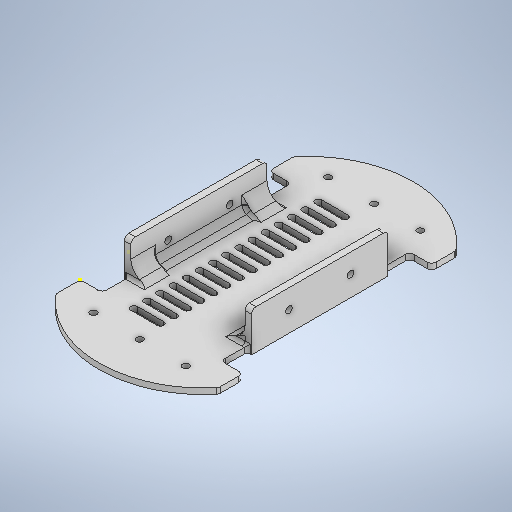
# Autodesk Inventor part: module_part2_nologo_asymmetric
Saved by Autodesk Inventor 2025.2 (Build 292293000, 293)
## iProperties
Created: 2025-05-02
Part Number: module_part2_nologo_asymmetric
Material: Generic
Document SubType Name: Modeling
Designer: holz
Density: 1 g/cm^3
Appearance: Default
Author: holz
Autodesk Inventor part; units mm, degrees
ref_plane "YZ Plane" through (0, 0, 0) normal (1, 0, 0) x (0, 1, 0)
ref_plane "XZ Plane" through (0, 0, 0) normal (0, 1, 0) x (-1, 0, 0)
ref_plane "XY Plane" through (0, 0, 0) normal (0, 0, 1) x (1, 0, 0)
sketch "Sketch1" plane through (0, 0, 0) normal (0, 1, 0) x (-1, 0, 0)
  line L0 (0, 0) -> (-74, 0)
  line L1 (-74, -86) -> (-74, -86)
  line L2 (-74, -86) -> (0, -86)
  line L3 (0, -86) -> (0, -97)
  line L4 (0, -97) -> (-74, -97)
  line L5 (-74, -97) -> (-74, -86)
  line L6 (-74, 0) -> (0, 0)
  line L7 (0, 0) -> (0, 11)
  line L8 (0, 11) -> (-74, 11)
  line L9 (-74, 11) -> (-74, 0)
  line L10 (-74, 11) -> (0, 11)
  line L11 (0, 11) -> (0, 28.5)
  line L12 (0, 28.5) -> (-74, 28.5)
  line L13 (-74, 28.5) -> (-74, 11)
  line L14 (-74, -97) -> (0, -97)
  line L15 (0, -97) -> (0, -114.5)
  line L16 (0, -114.5) -> (-74, -114.5)
  line L17 (-74, -114.5) -> (-74, -97)
  arc A0 (0, 11) -> (-74, 11) centre (-37, -19.3643) ccw
  arc A1 (-74, -97) -> (0, -97) centre (-37, -66.6357) ccw
  line L18 (-37, 0) -> (-65, 0)
  line L19 (-69, -86) -> (-39, -86)
  line L20 (-37, 0) -> (-5, 0)
  line L21 (-9, -86) -> (-39, -86)
  line L22 (-9, -86) -> (-10, -86)
  line L23 (-10, -86) -> (-10, 0)
  line L24 (-10, 0) -> (-8, 0)
  line L25 (-69, -86) -> (-66, -86)
  line L26 (-66, 0) -> (-65, 0)
  line L27 (0, 11) -> (-74, 11)
  line L28 (-74, 11) -> (-74, -49.7286)
  line L29 (-74, -49.7286) -> (0, -49.7286)
  line L30 (0, -49.7286) -> (0, 11)
  line L31 (-37, -49.7286) -> (-37, -97)
  line L32 (-37, -49.7286) -> (-37, 0)
  line L33 (-37, -97) -> (-10, -97)
  line L34 (-9, 0) -> (-37, 0)
  line L35 (-37, 0) -> (-37, -97)
  line L36 (-37, 0) -> (-64, 0)
  line L37 (-64, 0) -> (-64, -86)
  line L38 (-64, -86) -> (-37, -86)
  line L39 (-37, -86) -> (-37, 0)
  point P0 (-10, 0)
  dimension "d1" = 86
  dimension "d2" = 11
  dimension "d3" = 11
  dimension "d4" = 17.5
  dimension "d5" = 17.5
  dimension "d11" = 74
  dimension "d12" = 74
  dimension "d15" = 27
  dimension "d16" = 27
  constraints: 80 end point, 18 parallel, 12 horizontal, 8 point on line, 7 perpendicular, 6 point on circle, 5 midpoint, 2 centre point, 2 tangent, 1 collinear
  measures "d1" distance of L1.start L0.end
  measures "d2" distance of L2.end L3.end
  measures "d3" distance of L7.end L6.end
  measures "d4" distance of L11.end L10.end
  measures "d5" distance of L14.end L15.end
  measures "d11" distance of L7.end L8.end
  measures "d12" distance of L3.end L4.end
  measures "d15" distance of L23.end L36.start
  measures "d16" distance of L36.end L34.end
extrude "Extrusion1" add sketch "Sketch1" against normal blind 2.6 contours L0 L9 L8 L7 | L8 A0 | L29 L32 L0 L23 | L23 L2 L31 L29 | L2 L3 L4 L31 | L31 L2 L37 L29 | L29 L37 L0 L32 | L31 L4 L5 L2 | L4 A1
fillet "Face Fillet1" radius 2 1 edges at (74, -1.3, -86)
fillet "Face Fillet2" radius 2 1 edges at (64, -1.3, -86)
fillet "Face Fillet3" radius 2 1 edges at (74, -1.3, 11)
fillet "Face Fillet4" radius 2 1 edges at (0, -1.3, -86)
fillet "Face Fillet5" radius 2 1 edges at (0, -1.3, 11)
fillet "Face Fillet6" radius 2 1 edges at (0, -1.3, 0)
fillet "Face Fillet7" radius 2 1 edges at (0, -1.3, -97)
fillet "Face Fillet8" radius 2 1 edges at (74, -1.3, -97)
fillet "Face Fillet9" radius 2 1 edges at (74, -1.3, 0)
fillet "Face Fillet10" radius 2 1 edges at (10, -1.3, -86)
fillet "Face Fillet11" radius 2 1 edges at (10, -1.3, 0)
fillet "Face Fillet12" radius 2 1 edges at (64, -1.3, 0)
sketch "Sketch5" plane through (0, 0, 0) normal (0, 1, 0) x (1, 0, 0)
  arc A0 (10, 84) -> (8, 86) centre (8, 84) ccw projected
  line L0 (64, 2) -> (64, 84) projected
  line L1 (10, 84) -> (64, 84)
  line L2 (64, 84) -> (64, 71.4558)
  line L3 (64, 71.4558) -> (10, 71.4558)
  line L4 (10, 71.4558) -> (10, 84)
  line L5 (37, 84) -> (37, 60.4451)
  line L6 (26.2602, 84) -> (40.4168, 84)
  line L7 (40.4168, 84) -> (40.4168, 82.5)
  line L8 (40.4168, 82.5) -> (26.2602, 82.5)
  line L9 (26.2602, 82.5) -> (26.2602, 84)
  line L10 (8, 86) -> (2, 86) projected
  line L11 (2, 86) -> (74.2134, 86)
  line L12 (70.1915, 96.9) -> (-2.0219, 96.9)
  line L13 (70.1915, 96.9) -> (-4.0219, 96.9)
  line L14 (-4.0219, 96.9) -> (-4.0219, 86)
  line L15 (-4.0219, 86) -> (70.1915, 86)
  line L16 (74, 96.2758) -> (74, 88) projected
  line L17 (74, 88) -> (74, 85.5591)
  line L18 (74, 85.5591) -> (74, 96.9)
  line L19 (37, 84) -> (37, 116.0596)
  line L20 (37, 100.0298) -> (16, 100.0298)
  line L21 (16, 100.0298) -> (16, 86)
  line L22 (16, 86) -> (37, 86)
  line L23 (37, 86) -> (37, 100.0298)
  line L24 (37, 105.7284) -> (58, 105.7284)
  line L25 (58, 105.7284) -> (58, 86)
  line L26 (58, 86) -> (37, 86)
  line L27 (37, 86) -> (37, 105.7284)
  line L28 (16, 100.0298) -> (0, 100.0298)
  line L29 (0, 100.0298) -> (0, 86)
  line L30 (0, 86) -> (16, 86)
  line L31 (16, 86) -> (16, 100.0298)
  line L32 (58, 100.874) -> (74, 100.874)
  line L33 (74, 100.874) -> (74, 86)
  line L34 (74, 86) -> (58, 86)
  line L35 (58, 86) -> (58, 100.874)
  line L36 (10.4417, 86) -> (6.2096, 86)
  line L37 (6.2096, 86) -> (6.2096, 96.9)
  line L38 (6.2096, 96.9) -> (10.4417, 96.9)
  line L39 (10.4417, 96.9) -> (10.4417, 86)
  circle A1 centre (16, 96.9) radius 1.45
  circle A2 centre (37, 96.9) radius 1.45
  circle A3 centre (58, 96.9) radius 1.45
  line L40 (16, 96.9) -> (58, 96.9)
  line L41 (58, 96.9) -> (58, -18.2327)
  line L42 (58, -18.2327) -> (16, -18.2327)
  line L43 (16, -18.2327) -> (16, 96.9)
  line L44 (37, 100.0298) -> (37, -18.2327)
  line L45 (71.1847, 0) -> (5, 0)
  line L46 (5, 0) -> (5, -10)
  line L47 (5, -10) -> (71.1847, -10)
  line L48 (71.1847, -10) -> (71.1847, 0)
  circle A4 centre (58, -10) radius 1.5
  circle A5 centre (37, -10) radius 1.5
  circle A6 centre (16, -10) radius 1.5
  point P0 (0, 0)
  dimension "d63" = 1.5
  dimension "d65" = 21
  dimension "d66" = 21
  dimension "d67" = 10.9
  dimension "d68" = 2.9
  dimension "d69" = 2.9
  dimension "d70" = 2.9
  dimension "d71" = 10
  dimension "d72" = 3
  dimension "d73" = 3
  dimension "d74" = 3
  constraints: 92 end point, 25 point on line, 20 parallel, 11 horizontal, 10 perpendicular, 6 centre point, 3 midpoint, 3 vertical, 1 collinear
  measures "d63" distance of L7.end L6.end
  measures "d65" distance of L20.start L20.end
  measures "d66" distance of L24.start L24.end
  measures "d67" distance of L38.end L36.start
  measures "d68" diameter of A2
  measures "d69" diameter of A3
  measures "d70" diameter of A1
  measures "d71" distance of L45.end L46.end
  measures "d72" diameter of A6
  measures "d73" diameter of A5
  measures "d74" diameter of A4
sketch "Sketch6" plane through (0, 0, 0) normal (0, 1, 0) x (1, 0, 0)
  point P0 (0, 0)
sketch "Sketch8" plane through (64, -2.6, -84) normal (1, 0, 0) x (0, 0, -1)
  line L0 (-82, 0) -> (0, 0) projected
  line L1 (-82, 0) -> (0, 0)
  line L2 (0, 0) -> (0, 18)
  line L3 (0, 18) -> (-82, 18)
  line L4 (-82, 18) -> (-82, 0)
  line L5 (-82, 2.6) -> (0, 2.6) projected
  line L6 (-41, 0) -> (-41, 18)
  line L7 (-41, 18) -> (-72, 18)
  line L8 (-72, 18) -> (-72, 0)
  line L9 (-72, 0) -> (-41, 0)
  line L10 (-41, 0) -> (-41, 18)
  line L11 (-41, 18) -> (-10, 18)
  line L12 (-10, 18) -> (-10, 0)
  line L13 (-10, 0) -> (-41, 0)
  line L14 (-41, 0) -> (-41, 18)
  point P0 (-84, 2.6)
  point P1 (-72, 0)
  point P2 (-10, 0)
  point P3 (-10, 18)
  dimension "d87" = 18
  dimension "d88" = 82
  dimension "d89" = 31
  dimension "d90" = 31
  constraints: 26 end point, 7 parallel, 3 perpendicular, 2 horizontal, 2 midpoint, 2 point on line
  measures "d87" distance of L1.end L2.end
  measures "d88" distance of L2.end L3.end
  measures "d89" distance of L6.end L11.end
  measures "d90" distance of L7.end L6.end
sketch "Sketch9" plane through (10, -2.6, -84) normal (-1, 0, 0) x (0, 0, 1)
  line L0 (0, 2.6) -> (0, 0) projected
  line L1 (0, 0) -> (72.0022, 0)
  line L2 (72.0022, 0) -> (72.0022, 18)
  line L3 (72.0022, 18) -> (0, 18)
  line L4 (0, 18) -> (0, 0)
  line L5 (82, 2.6) -> (0, 2.6) projected
  line L6 (41, 2.6) -> (10, 2.6)
  line L7 (10, 2.6) -> (10, 18)
  line L8 (10, 18) -> (41, 18)
  line L9 (41, 18) -> (41, 2.6)
  line L10 (72.0022, 18) -> (10, 18)
  line L11 (10, 18) -> (10, 0)
  line L12 (10, 0) -> (72.0022, 0)
  line L13 (72.0022, 0) -> (72.0022, 18)
  point P0 (84, 2.6)
  point P1 (10, 18)
  point P2 (10, 2.6)
  dimension "d91" = 31
  dimension "d92" = 18
  constraints: 24 end point, 6 parallel, 3 horizontal, 3 perpendicular, 1 midpoint, 1 point on line
  measures "d91" distance of L7.end L8.end
  measures "d92" distance of L10.end L11.end
extrude "Extrusion5" add sketch "Sketch8" along normal blind 2 contours L8 L5 L6 L0 | L6 L5 L12 L0 | L8 L3 L6 L5 | L6 L3 L12 L5
extrude "Extrusion6" add sketch "Sketch9" along normal blind 2 contours L7 L3 L9 L5 | L5 L2 L1 L11 | L9 L3 L2 L5
sketch "Sketch10" plane through (10, -2.6, -84) normal (1, 0, 0) x (0, 0, -1)
  line L0 (-72.0022, 0) -> (-72.0022, 18) projected
  line L1 (-72.0022, 18) -> (-10, 18)
  line L2 (-10, 18) -> (-10, 2.1531)
  line L3 (-10, 2.1531) -> (-72.0022, 2.1531)
  line L4 (-72.0022, 2.1531) -> (-72.0022, 18)
  point P0 (-84, 2.6)
  constraints: 8 end point, 2 parallel, 1 horizontal, 1 perpendicular
extrude "Extrusion7" add sketch "Sketch10" along normal blind 1
sketch "Sketch11" plane through (64, -2.6, -84) normal (-1, 0, 0) x (0, 0, 1)
  line L0 (10, 0) -> (10, 18) projected
  line L1 (72, 2.6) -> (10, 2.6) projected
  line L2 (10, 18) -> (72, 18)
  line L3 (72, 18) -> (72, 2.6)
  line L4 (72, 2.6) -> (10, 2.6)
  line L5 (10, 2.6) -> (10, 18)
  point P0 (84, 2.6)
  constraints: 8 end point, 2 parallel, 1 horizontal, 1 perpendicular
extrude "Extrusion8" add sketch "Sketch11" along normal blind 1
sketch "Sketch13" plane through (66, -2.6, -84) normal (1, 0, 0) x (0, 0, -1)
  line L0 (-10, 0) -> (-72.0022, 0) projected
  line L1 (-41.0011, 0) -> (-41.0011, 18)
  line L2 (-10, 18) -> (-72.0022, 18) projected
  line L3 (-41.0011, 18) -> (-55.0011, 18)
  line L4 (-55.0011, 18) -> (-55.0011, 0)
  line L5 (-55.0011, 0) -> (-41.0011, 0)
  line L6 (-41.0011, 0) -> (-41.0011, 18)
  line L7 (-41.0011, 18) -> (-27.0011, 18)
  line L8 (-27.0011, 18) -> (-27.0011, 0)
  line L9 (-27.0011, 0) -> (-41.0011, 0)
  line L10 (-41.0011, 0) -> (-41.0011, 18)
  line L11 (-55.0011, 0) -> (-58.5071, 0)
  line L12 (-58.5071, 0) -> (-58.5071, 9.3)
  line L13 (-58.5071, 9.3) -> (-55.0011, 9.3)
  line L14 (-55.0011, 9.3) -> (-55.0011, 0)
  line L15 (-27.0011, 0) -> (-20.3269, 0)
  line L16 (-20.3269, 0) -> (-20.3269, 9.3)
  line L17 (-20.3269, 9.3) -> (-27.0011, 9.3)
  line L18 (-27.0011, 9.3) -> (-27.0011, 0)
  circle A0 centre (-55.0011, 9.3) radius 1.5
  circle A1 centre (-27.0011, 9.3) radius 1.5
  point P0 (-84, 2.6)
  dimension "d101" = 14
  dimension "d102" = 14
  dimension "d103" = 18
  dimension "d104" = 9.3
  dimension "d105" = 9.3
  dimension "d106" = 3
  dimension "d107" = 3
  constraints: 34 end point, 8 parallel, 4 horizontal, 4 perpendicular, 2 centre point, 2 coincident, 2 midpoint, 2 point on line
  measures "d101" distance of L1.end L3.end
  measures "d102" distance of L7.end L1.end
  measures "d103" distance of L3.end L4.end
  measures "d104" distance of L11.end L12.end
  measures "d105" distance of L15.end L16.end
  measures "d106" diameter of A0
  measures "d107" diameter of A1
sketch "Sketch14" plane through (8, -2.6, -84) normal (-1, 0, 0) x (0, 0, 1)
  circle A0 centre (55.0011, 9.3) radius 1.5
  circle A1 centre (27.0011, 9.3) radius 1.5
  point P0 (84, 2.6)
  dimension "d108" = 3
  dimension "d109" = 3
  constraints: 2 centre point
  measures "d108" diameter of A0
  measures "d109" diameter of A1
extrude "Extrusion9" cut sketch "Sketch13" along normal mid plane 40 contours A1 L8 | L8 L17 A1 | L17 L8 A1 | A0 L13 L4 | L4 A0 | L13 A0 L4
extrude "Extrusion10" cut sketch "Sketch14" against normal blind 40
fillet "Face Fillet13" radius 2 1 edges at (64.5, 15.4, -12)
fillet "Face Fillet14" radius 2 2 edges at (9, 15.4, -11.9978) (10.5, 15.4, -11.9978)
fillet "Face Fillet15" radius 2 1 edges at (64.5, 15.4, -74)
fillet "Face Fillet16" radius 2 2 edges at (10.5, 15.4, -74) (9, 15.4, -74)
extrude "Extrusion12" cut sketch "Sketch5" against normal blind 10 contours A1 L12 L21 | L21 L12 A1 | A1 L21 L12 | A6 L47 L43 | L43 L47 A6 | A2 L12 L19 | L19 L12 A2 | L21 A1 L12 | L47 A6 L43 | L43 A6 L47 | A5 L47 L44 | L44 L47 A5 | A3 L12 L25 | L25 L12 A3 | L19 A2 L12 | L12 A2 L19 | A4 L47 L41 | L41 L47 A4 | L47 L44 A5 | L47 A5 L44 | L25 A3 L12 | L12 A3 L25 | L47 A4 L41 | L41 A4 L47
sketch "Sketch15" plane through (0, 0, 0) normal (0, 1, 0) x (1, 0, 0)
  arc A0 (8, 0) -> (10, 2) centre (8, 2) ccw projected
  line L0 (66, 0) -> (66, 86)
  line L1 (8, 86) -> (8, 0)
  line L2 (66.8194, 0) -> (66.8194, -0.5)
  line L3 (66.8194, -0.5) -> (0, -0.5)
  line L4 (0, -0.5) -> (0, 0)
  line L5 (72.054, 86) -> (72.054, 86.5)
  line L6 (72.054, 86.5) -> (8, 86.5)
  line L7 (8, 86.5) -> (8, 86)
  line L8 (10, 2) -> (10, 11.9978) projected
  line L9 (22, 2) -> (22, 89.1821)
  line L10 (22, 89.1821) -> (10, 89.1821)
  line L11 (10, 89.1821) -> (10, 2)
  line L12 (10, 2) -> (10, -16.2601)
  line L13 (10, -16.2601) -> (22, -16.2601)
  line L14 (22, -16.2601) -> (22, 2)
  line L15 (22, 86.5) -> (37, 86.5)
  line L16 (37, 86.5) -> (37, -0.5)
  line L17 (37, -0.5) -> (22, -0.5)
  line L18 (22, -0.5) -> (22, 86.5)
  line L19 (22, -0.5) -> (37, -0.5)
  line L20 (37, -0.5) -> (37, 2.5)
  line L21 (37, 2.5) -> (22, 2.5)
  line L22 (22, 2.5) -> (22, -0.5)
  line L23 (22, 2.5) -> (37, 2.5)
  line L24 (37, 2.5) -> (37, 5.5)
  line L25 (37, 5.5) -> (22, 5.5)
  line L26 (22, 5.5) -> (22, 2.5)
  line L27 (22, 5.5) -> (37, 5.5)
  line L28 (37, 5.5) -> (37, 8.5)
  line L29 (37, 8.5) -> (22, 8.5)
  line L30 (22, 8.5) -> (22, 5.5)
  line L31 (22, 8.5) -> (37, 8.5)
  line L32 (37, 8.5) -> (37, 11.5)
  line L33 (37, 11.5) -> (22, 11.5)
  line L34 (22, 11.5) -> (22, 8.5)
  line L35 (22, 11.5) -> (37, 11.5)
  line L36 (37, 11.5) -> (37, 14.5)
  line L37 (37, 14.5) -> (22, 14.5)
  line L38 (22, 14.5) -> (22, 11.5)
  line L39 (22, 14.5) -> (37, 14.5)
  line L40 (37, 14.5) -> (37, 17.5)
  line L41 (37, 17.5) -> (22, 17.5)
  line L42 (22, 17.5) -> (22, 14.5)
  line L43 (22, 17.5) -> (37, 17.5)
  line L44 (37, 17.5) -> (37, 20.5)
  line L45 (37, 20.5) -> (22, 20.5)
  line L46 (22, 20.5) -> (22, 17.5)
  line L47 (22, 20.5) -> (37, 20.5)
  line L48 (37, 20.5) -> (37, 23.5)
  line L49 (37, 23.5) -> (22, 23.5)
  line L50 (22, 23.5) -> (22, 20.5)
  line L51 (22, 23.5) -> (37, 23.5)
  line L52 (37, 23.5) -> (37, 80.5)
  line L53 (37, 80.5) -> (22, 80.5)
  line L54 (22, 80.5) -> (22, 23.5)
  line L55 (22, 80.5) -> (37, 80.5)
  line L56 (37, 80.5) -> (37, 83.5)
  line L57 (37, 83.5) -> (22, 83.5)
  line L58 (22, 83.5) -> (22, 80.5)
  line L59 (22, 23.5) -> (37, 23.5)
  line L60 (37, 23.5) -> (37, 26.5)
  line L61 (37, 26.5) -> (22, 26.5)
  line L62 (22, 26.5) -> (22, 23.5)
  line L63 (22, 26.5) -> (37, 26.5)
  line L64 (37, 26.5) -> (37, 29.5)
  line L65 (37, 29.5) -> (22, 29.5)
  line L66 (22, 29.5) -> (22, 26.5)
  line L67 (22, 29.5) -> (37, 29.5)
  line L68 (37, 29.5) -> (37, 32.5)
  line L69 (37, 32.5) -> (22, 32.5)
  line L70 (22, 32.5) -> (22, 29.5)
  line L71 (22, 32.5) -> (37, 32.5)
  line L72 (37, 32.5) -> (37, 35.5)
  line L73 (37, 35.5) -> (22, 35.5)
  line L74 (22, 35.5) -> (22, 32.5)
  line L75 (22, 35.5) -> (37, 35.5)
  line L76 (37, 35.5) -> (37, 38.5)
  line L77 (37, 38.5) -> (22, 38.5)
  line L78 (22, 38.5) -> (22, 35.5)
  line L79 (22, 38.5) -> (37, 38.5)
  line L80 (37, 38.5) -> (37, 41.5)
  line L81 (37, 41.5) -> (22, 41.5)
  line L82 (22, 41.5) -> (22, 38.5)
  line L83 (22, 41.5) -> (37, 41.5)
  line L84 (37, 41.5) -> (37, 44.5)
  line L85 (37, 44.5) -> (22, 44.5)
  line L86 (22, 44.5) -> (22, 41.5)
  line L87 (22, 44.5) -> (37, 44.5)
  line L88 (37, 44.5) -> (37, 77.5)
  line L89 (37, 77.5) -> (22, 77.5)
  line L90 (22, 77.5) -> (22, 44.5)
  line L91 (22, 44.5) -> (37, 44.5)
  line L92 (37, 44.5) -> (37, 47.5)
  line L93 (37, 47.5) -> (22, 47.5)
  line L94 (22, 47.5) -> (22, 44.5)
  line L95 (22, 47.5) -> (37, 47.5)
  line L96 (37, 47.5) -> (37, 50.5)
  line L97 (37, 50.5) -> (22, 50.5)
  line L98 (22, 50.5) -> (22, 47.5)
  line L99 (22, 50.5) -> (37, 50.5)
  line L100 (37, 50.5) -> (37, 53.5)
  line L101 (37, 53.5) -> (22, 53.5)
  line L102 (22, 53.5) -> (22, 50.5)
  line L103 (22, 53.5) -> (37, 53.5)
  line L104 (37, 53.5) -> (37, 56.5)
  line L105 (37, 56.5) -> (22, 56.5)
  line L106 (22, 56.5) -> (22, 53.5)
  line L107 (22, 56.5) -> (37, 56.5)
  line L108 (37, 56.5) -> (37, 71.5)
  line L109 (37, 71.5) -> (22, 71.5)
  line L110 (22, 71.5) -> (22, 56.5)
  line L111 (22, 71.5) -> (37, 71.5)
  line L112 (37, 71.5) -> (37, 74.5)
  line L113 (37, 74.5) -> (22, 74.5)
  line L114 (22, 74.5) -> (22, 71.5)
  line L115 (22, 56.5) -> (37, 56.5)
  line L116 (37, 56.5) -> (37, 59.5)
  line L117 (37, 59.5) -> (22, 59.5)
  line L118 (22, 59.5) -> (22, 56.5)
  line L119 (22, 59.5) -> (37, 59.5)
  line L120 (37, 59.5) -> (37, 62.5)
  line L121 (37, 62.5) -> (22, 62.5)
  line L122 (22, 62.5) -> (22, 59.5)
  line L123 (22, 62.5) -> (37, 62.5)
  line L124 (37, 62.5) -> (37, 65.5)
  line L125 (37, 65.5) -> (22, 65.5)
  line L126 (22, 65.5) -> (22, 62.5)
  line L127 (22, 65.5) -> (37, 65.5)
  line L128 (37, 65.5) -> (37, 68.5)
  line L129 (37, 68.5) -> (22, 68.5)
  line L130 (22, 68.5) -> (22, 65.5)
  line L131 (22, 68.5) -> (37, 68.5)
  line L132 (37, 68.5) -> (37, 71.5)
  line L133 (37, 71.5) -> (22, 71.5)
  line L134 (22, 71.5) -> (22, 68.5)
  line L135 (37, 73) -> (22, 73)
  line L136 (37, 86.5) -> (22, 86.5)
  line L137 (22, 86.5) -> (22, 85)
  line L138 (22, 85) -> (37, 85)
  line L139 (37, 85) -> (37, 86.5)
  line L140 (37, 80.5) -> (22, 80.5)
  line L141 (22, 80.5) -> (22, 79)
  line L142 (22, 79) -> (37, 79)
  line L143 (37, 79) -> (37, 80.5)
  line L144 (37, 67) -> (22, 67)
  line L145 (22, 67) -> (22, 65.5)
  line L146 (22, 65.5) -> (37, 65.5)
  line L147 (37, 65.5) -> (37, 67)
  line L148 (37, 61) -> (22, 61)
  line L149 (22, 61) -> (22, 59.5)
  line L150 (22, 59.5) -> (37, 59.5)
  line L151 (37, 59.5) -> (37, 61)
  line L152 (37, 55) -> (22, 55)
  line L153 (22, 55) -> (22, 53.5)
  line L154 (22, 53.5) -> (37, 53.5)
  line L155 (37, 53.5) -> (37, 55)
  line L156 (37, 49) -> (22, 49)
  line L157 (22, 49) -> (22, 50.5)
  line L158 (22, 50.5) -> (37, 50.5)
  line L159 (37, 50.5) -> (37, 49)
  line L160 (37, 43) -> (22, 43)
  line L161 (22, 43) -> (22, 41.5)
  line L162 (22, 41.5) -> (37, 41.5)
  line L163 (37, 41.5) -> (37, 43)
  line L164 (37, 37) -> (22, 37)
  line L165 (22, 37) -> (22, 35.5)
  line L166 (22, 35.5) -> (37, 35.5)
  line L167 (37, 35.5) -> (37, 37)
  line L168 (37, 31) -> (22, 31)
  line L169 (22, 31) -> (22, 29.5)
  line L170 (22, 29.5) -> (37, 29.5)
  line L171 (37, 29.5) -> (37, 31)
  line L172 (37, 25) -> (22, 25)
  line L173 (22, 25) -> (22, 23.5)
  line L174 (22, 23.5) -> (37, 23.5)
  line L175 (37, 23.5) -> (37, 25)
  line L176 (37, 19) -> (22, 19)
  line L177 (22, 19) -> (22, 17.5)
  line L178 (22, 17.5) -> (37, 17.5)
  line L179 (37, 17.5) -> (37, 19)
  line L180 (37, 13) -> (22, 13)
  line L181 (22, 13) -> (22, 11.5)
  line L182 (22, 11.5) -> (37, 11.5)
  line L183 (37, 11.5) -> (37, 13)
  line L184 (37, 7) -> (22, 7)
  line L185 (22, 7) -> (22, 5.5)
  line L186 (22, 5.5) -> (37, 5.5)
  line L187 (37, 5.5) -> (37, 7)
  line L188 (37, 1) -> (22, 1)
  line L189 (22, 1) -> (22, 2.5)
  line L190 (22, 2.5) -> (37, 2.5)
  line L191 (37, 2.5) -> (37, 1)
  line L192 (37, 86.5) -> (23.5, 86.5)
  line L193 (23.5, 86.5) -> (23.5, -0.5)
  line L194 (23.5, -0.5) -> (37, -0.5)
  line L195 (37, -0.5) -> (37, 86.5)
  line L196 (22, 86.5) -> (35.5, 86.5)
  line L197 (35.5, 86.5) -> (35.5, -0.5)
  line L198 (35.5, -0.5) -> (22, -0.5)
  line L199 (22, -0.5) -> (22, 86.5)
  line L200 (35.5, 85) -> (23.5, 85) construction
  line L201 (35.5, 86.5) -> (23.5, 86.5)
  line L202 (23.5, 83.5) -> (35.5, 83.5)
  arc A1 (35.5, 83.5) -> (35.5, 86.5) centre (35.5, 85) ccw
  arc A2 (23.5, 86.5) -> (23.5, 83.5) centre (23.5, 85) ccw
  line L203 (35.5, 79) -> (23.5, 79) construction
  line L204 (35.5, 73) -> (23.5, 73) construction
  line L205 (35.5, 74.5) -> (23.5, 74.5)
  line L206 (23.5, 71.5) -> (35.5, 71.5)
  arc A3 (35.5, 71.5) -> (35.5, 74.5) centre (35.5, 73) ccw
  arc A4 (23.5, 74.5) -> (23.5, 71.5) centre (23.5, 73) ccw
  line L207 (35.5, 67) -> (23.5, 67) construction
  line L208 (35.5, 68.5) -> (23.5, 68.5)
  line L209 (23.5, 65.5) -> (35.5, 65.5)
  arc A5 (35.5, 65.5) -> (35.5, 68.5) centre (35.5, 67) ccw
  arc A6 (23.5, 68.5) -> (23.5, 65.5) centre (23.5, 67) ccw
  line L210 (35.5, 61) -> (23.5, 61) construction
  line L211 (35.5, 62.5) -> (23.5, 62.5)
  line L212 (23.5, 59.5) -> (35.5, 59.5)
  arc A7 (35.5, 59.5) -> (35.5, 62.5) centre (35.5, 61) ccw
  arc A8 (23.5, 62.5) -> (23.5, 59.5) centre (23.5, 61) ccw
  line L213 (35.5, 55) -> (23.5, 55) construction
  line L214 (35.5, 56.5) -> (23.5, 56.5)
  line L215 (23.5, 53.5) -> (35.5, 53.5)
  arc A9 (35.5, 53.5) -> (35.5, 56.5) centre (35.5, 55) ccw
  arc A10 (23.5, 56.5) -> (23.5, 53.5) centre (23.5, 55) ccw
  line L216 (35.5, 49) -> (23.5, 49) construction
  line L217 (35.5, 50.5) -> (23.5, 50.5)
  line L218 (23.5, 47.5) -> (35.5, 47.5)
  arc A11 (35.5, 47.5) -> (35.5, 50.5) centre (35.5, 49) ccw
  arc A12 (23.5, 50.5) -> (23.5, 47.5) centre (23.5, 49) ccw
  line L219 (35.5, 43) -> (23.5, 43) construction
  line L220 (35.5, 44.5) -> (23.5, 44.5)
  line L221 (23.5, 41.5) -> (35.5, 41.5)
  arc A13 (35.5, 41.5) -> (35.5, 44.5) centre (35.5, 43) ccw
  arc A14 (23.5, 44.5) -> (23.5, 41.5) centre (23.5, 43) ccw
  line L222 (35.5, 37) -> (23.5, 37) construction
  line L223 (35.5, 38.5) -> (23.5, 38.5)
  line L224 (23.5, 35.5) -> (35.5, 35.5)
  arc A15 (35.5, 35.5) -> (35.5, 38.5) centre (35.5, 37) ccw
  arc A16 (23.5, 38.5) -> (23.5, 35.5) centre (23.5, 37) ccw
  line L225 (35.5, 31) -> (23.5, 31) construction
  line L226 (35.5, 29.5) -> (23.5, 29.5)
  line L227 (23.5, 32.5) -> (35.5, 32.5)
  arc A17 (35.5, 29.5) -> (35.5, 32.5) centre (35.5, 31) ccw
  arc A18 (23.5, 32.5) -> (23.5, 29.5) centre (23.5, 31) ccw
  line L228 (35.5, 25) -> (23.5, 25) construction
  line L229 (35.5, 26.5138) -> (23.5, 26.5138)
  line L230 (23.5, 23.4862) -> (35.5, 23.4862)
  arc A19 (35.5, 23.4862) -> (35.5, 26.5138) centre (35.5, 25) ccw
  arc A20 (23.5, 26.5138) -> (23.5, 23.4862) centre (23.5, 25) ccw
  line L231 (35.5, 19) -> (23.5, 19) construction
  line L232 (35.5, 20.5) -> (23.5, 20.5)
  line L233 (23.5, 17.5) -> (35.5, 17.5)
  arc A21 (35.5, 17.5) -> (35.5, 20.5) centre (35.5, 19) ccw
  arc A22 (23.5, 20.5) -> (23.5, 17.5) centre (23.5, 19) ccw
  line L234 (35.5, 13) -> (23.5, 13) construction
  line L235 (35.5, 14.5) -> (23.5, 14.5)
  line L236 (23.5, 11.5) -> (35.5, 11.5)
  arc A23 (35.5, 11.5) -> (35.5, 14.5) centre (35.5, 13) ccw
  arc A24 (23.5, 14.5) -> (23.5, 11.5) centre (23.5, 13) ccw
  line L237 (35.5, 7) -> (23.5, 7) construction
  line L238 (35.5, 8.5) -> (23.5, 8.5)
  line L239 (23.5, 5.5) -> (35.5, 5.5)
  arc A25 (35.5, 5.5) -> (35.5, 8.5) centre (35.5, 7) ccw
  arc A26 (23.5, 8.5) -> (23.5, 5.5) centre (23.5, 7) ccw
  line L240 (35.5, 1) -> (23.5, 1) construction
  line L241 (35.5, -0.5) -> (23.5, -0.5)
  line L242 (23.5, 2.5) -> (35.5, 2.5)
  arc A27 (35.5, -0.5) -> (35.5, 2.5) centre (35.5, 1) ccw
  arc A28 (23.5, 2.5) -> (23.5, -0.5) centre (23.5, 1) ccw
  line L243 (35.5, 79) -> (23.5, 79) construction
  line L244 (35.5, 80.5) -> (23.5, 80.5)
  line L245 (23.5, 77.5) -> (35.5, 77.5)
  arc A29 (35.5, 77.5) -> (35.5, 80.5) centre (35.5, 79) ccw
  arc A30 (23.5, 80.5) -> (23.5, 77.5) centre (23.5, 79) ccw
  point P0 (22, -0.5)
  point P1 (29.5, 85)
  point P2 (29.5, 79)
  point P3 (29.5, 73)
  point P4 (29.5, 67)
  point P5 (29.5, 61)
  point P6 (29.5, 55)
  point P7 (29.5, 49)
  point P8 (29.5, 43)
  point P9 (29.5, 37)
  point P10 (29.5, 31)
  point P11 (29.5, 25)
  point P12 (29.5, 19)
  point P13 (29.5, 13)
  point P14 (29.5, 7)
  point P15 (29.5, 1)
  point P16 (29.5, 79)
  point P17 (35.5, -0.5)
  point P18 (35.5, 2.5)
  point P19 (23.5, 2.5)
  point P20 (23.5, -0.5)
  point P21 (35.5, 8.5)
  point P22 (23.5, 8.5)
  point P23 (23.5, 5.5)
  point P24 (35.5, 14.5)
  point P25 (23.5, 14.5)
  point P26 (23.5, 20.5)
  point P27 (35.5, 20.5)
  point P28 (35.7039, 23.5)
  point P29 (37, 24.7961)
  point P30 (37, 25.2039)
  point P31 (35.7039, 26.5)
  point P32 (23.2961, 26.5)
  point P33 (22, 25.2039)
  point P34 (22, 24.7961)
  point P35 (23.2961, 23.5)
  point P36 (23.5, 29.5)
  point P37 (23.5, 38.5)
  point P38 (23.5, 35.5)
  point P39 (35.5, 35.5)
  point P40 (35.5, 38.5)
  point P41 (23.5, 44.5)
  point P42 (35.5, 44.5)
  point P43 (23.5, 50.5)
  point P44 (23.5, 47.5)
  point P45 (35.5, 50.5)
  point P46 (23.5, 56.5)
  point P47 (35.5, 56.5)
  point P48 (23.5, 62.5)
  point P49 (35.5, 59.5)
  point P50 (35.5, 62.5)
  point P51 (23.5, 68.5)
  point P52 (35.5, 65.5)
  point P53 (35.5, 68.5)
  point P54 (23.5, 71.5)
  point P55 (35.5, 74.5)
  point P56 (35.5, 77.5)
  point P57 (35.5, 80.5)
  point P58 (23.5, 80.5)
  point P59 (35.5, 29.5)
  dimension "d125" = 86
  dimension "d126" = 0.5
  dimension "d127" = 0.5
  dimension "d128" = 12
  dimension "d129" = 15
  dimension "d130" = 3
  dimension "d131" = 3
  dimension "d132" = 3
  dimension "d133" = 3
  dimension "d134" = 3
  dimension "d135" = 3
  dimension "d136" = 3
  dimension "d137" = 3
  dimension "d138" = 3
  dimension "d139" = 3
  dimension "d140" = 3
  dimension "d141" = 3
  dimension "d142" = 3
  dimension "d143" = 3
  dimension "d144" = 3
  dimension "d145" = 3
  dimension "d146" = 3
  dimension "d147" = 3
  dimension "d148" = 3
  dimension "d149" = 3
  dimension "d150" = 3
  dimension "d151" = 3
  dimension "d152" = 3
  dimension "d153" = 3
  dimension "d154" = 3
  dimension "d155" = 3
  dimension "d156" = 3
  dimension "d157" = 3
  dimension "d158" = 3
  dimension "d163" = 1.5
  dimension "d164" = 1.5
  dimension "d165" = 13.5
  dimension "d166" = 13.5
  constraints: 512 end point, 107 parallel, 61 point on circle, 60 tangent, 51 horizontal, 44 point on line, 42 perpendicular, 30 centre point, 30 midpoint, 5 vertical, 64 other
  measures "d125" distance of L1.start L1.end
  measures "d126" distance of L2.end L2.start
  measures "d127" distance of L5.end L5.start
  measures "d128" distance of L10.start L10.end
  measures "d129" distance of L15.start L15.end
  measures "d130" distance of L17.start L20.end
  measures "d131" distance of L20.end L24.end
  measures "d132" distance of L28.end L24.end
  measures "d133" distance of L32.end L28.end
  measures "d134" distance of L36.end L32.end
  measures "d135" distance of L40.end L36.end
  measures "d136" distance of L47.end L40.end
  measures "d137" distance of L47.end L48.end
  measures "d138" distance of L15.end L56.end
  measures "d139" distance of L56.end L53.start
  measures "d140" distance of L60.end L59.end
  measures "d141" distance of L64.end L60.end
  measures "d142" distance of L68.end L64.end
  measures "d143" distance of L75.end L68.end
  measures "d144" distance of L76.end L72.end
  measures "d145" distance of L80.end L76.end
  measures "d146" distance of L84.end L83.end
  measures "d147" distance of L53.start L88.end
  measures "d148" distance of L84.end L92.end
  measures "d149" distance of L92.end L96.end
  measures "d150" distance of L96.end L100.end
  measures "d151" distance of L100.end L104.end
  measures "d152" distance of L88.end L112.end
  measures "d153" distance of L112.end L108.end
  measures "d154" distance of L116.end L104.end
  measures "d155" distance of L123.end L116.end
  measures "d156" distance of L123.end L127.end
  measures "d157" distance of L124.end L128.end
  measures "d158" distance of L108.end L128.end
  measures "d163" distance of L136.end L137.end
  measures "d164" distance of L53.end L141.end
  measures "d165" distance of L15.end L192.end
  measures "d166" distance of L17.end L198.start
extrude "Extrusion14" cut sketch "Sketch15" along normal mid plane 40 contours L193 L188 L197 L3 | A28 L188 L193 | A28 L193 L188 | L6 L197 L138 L193 | L193 L138 A2 | L138 L193 A2 | L197 L188 A27 | L193 L21 L197 L188 | A1 L138 L197 | L138 L197 L57 L193 | L197 A27 L188 | L193 L184 L197 L25 | A26 L184 L193 | L138 A1 L197 | L53 L197 L142 L193 | L193 L142 A30 | L197 L184 A25 | L193 L29 L197 L184 | L184 A26 L193 | L142 L193 A30 | A29 L142 L197 | L142 L197 L89 L193 | L197 A25 L184 | L142 A29 L197 | L193 L180 L197 L33 | A24 L180 L193 | L113 L197 L135 L193 | L193 L135 A4 | L197 L180 A23 | L193 L37 L197 L180 | L180 A24 L193 | L135 L193 A4 | A3 L135 L197 | L135 L197 L109 L193 | L197 A23 L180 | L135 A3 L197 | L193 L176 L197 L41 | A22 L176 L193 | L129 L197 L144 L193 | L193 L144 A6 | L197 L176 A21 | L193 L45 L197 L176 | L176 A22 L193 | L144 L193 A6 | A5 L144 L197 | L144 L197 L125 L193 | L197 A21 L176 | L144 A5 L197 | L121 L197 L148 L193 | L193 L148 A8 | L193 L172 L197 L49 | L49 A20 L9 L172 L193 | L148 L193 A8 | A7 L148 L197 | L148 L197 L117 L193 | L197 L172 L16 A19 L49 | L193 L61 L197 L172 | L172 L9 A20 L61 L193 | L148 A7 L197 | L197 L61 A19 L16 L172 | L105 L197 L152 L193 | L193 L152 A10 | L152 L193 A10 | A9 L152 L197 | L152 L197 L101 L193 | L193 L168 L197 L65 | A18 L168 L193 | A18 L193 L168 | L152 A9 L197 | L197 L168 A17 | L168 L197 A17 | L193 L69 L197 L168 | L97 L197 L156 L193 | L193 L156 A12 | L193 L164 L197 L73 | A16 L164 L193 | L156 L193 A12 | A11 L156 L197 | L156 L197 L93 L193 | L197 L164 A15 | A16 L193 L164 | L193 L77 L197 L164 | L156 A11 L197 | L164 L197 A15 | L85 L197 L160 L193 | L193 L160 A14 | L193 L160 L197 L81 | A14 L160 L193 | A13 L160 L197 | L197 L160 A13
sketch "Sketch16" plane through (10, -2.6, -11.9978) normal (0, 0, 1) x (1, 0, 0)
  line L0 (1, 16) -> (1, 2.6) projected
  line L1 (-2, 16) -> (1, 16) projected
  line L2 (1, 2.6) -> (-0.5, 2.6)
  line L3 (-0.5, 2.6) -> (-0.5, 16)
  line L4 (-0.5, 16) -> (1, 16)
  line L5 (1, 16) -> (1, 2.6)
  line L6 (53, 2.6) -> (54.5, 2.6)
  line L7 (54.5, 2.6) -> (54.5, 16)
  line L8 (54.5, 16) -> (53, 16)
  line L9 (53, 16) -> (53, 2.6)
  line L10 (-0.5, 2.6) -> (8.5, 2.6)
  line L11 (8.5, 2.6) -> (8.5, 6.6)
  line L12 (8.5, 6.6) -> (-0.5, 6.6)
  line L13 (-0.5, 6.6) -> (-0.5, 2.6)
  line L14 (54.5, 2.6) -> (45.5, 2.6)
  line L15 (45.5, 2.6) -> (45.5, 6.6)
  line L16 (45.5, 6.6) -> (54.5, 6.6)
  line L17 (54.5, 6.6) -> (54.5, 2.6)
  line L18 (-0.5, 6.6) -> (8.5, 2.6)
  line L19 (54.5, 6.6) -> (45.5, 2.6)
  point P0 (-10, 2.6)
  point P1 (1, 5.9333)
  point P2 (53, 5.9333)
  dimension "d167" = 1.5
  dimension "d168" = 1.5
  dimension "d169" = 9
  dimension "d170" = 4
  dimension "d171" = 9
  dimension "d172" = 4
  constraints: 36 end point, 8 parallel, 4 horizontal, 4 perpendicular, 2 point on line, 1 midpoint
  measures "d167" distance of L3.end L4.end
  measures "d168" distance of L8.end L7.end
  measures "d169" distance of L12.end L11.end
  measures "d170" distance of L11.end L10.end
  measures "d171" distance of L15.end L16.end
  measures "d172" distance of L14.end L15.end
sketch "Sketch17" plane through (64, -2.6, -74) normal (0, 0, -1) x (-1, 0, 0)
  line L0 (0, 2.6) -> (1, 2.6) projected
  line L1 (1, 2.6) -> (-0.5, 2.6)
  line L2 (-0.5, 2.6) -> (-0.5, 6.6)
  line L3 (-0.5, 6.6) -> (1, 6.6)
  line L4 (1, 6.6) -> (1, 2.6)
  line L5 (53, 16) -> (53, 2.6) projected
  line L6 (53, 2.6) -> (54.5, 2.6)
  line L7 (54.5, 2.6) -> (54.5, 6.6)
  line L8 (54.5, 6.6) -> (53, 6.6)
  line L9 (53, 6.6) -> (53, 2.6)
  line L10 (54.5, 2.6) -> (45.5, 2.6)
  line L11 (45.5, 2.6) -> (45.5, 6.6)
  line L12 (45.5, 6.6) -> (54.5, 6.6)
  line L13 (54.5, 6.6) -> (54.5, 2.6)
  line L14 (54.5, 6.6) -> (45.5, 2.6)
  line L15 (-0.5, 2.6) -> (8.5, 2.6)
  line L16 (8.5, 2.6) -> (8.5, 6.6)
  line L17 (8.5, 6.6) -> (-0.5, 6.6)
  line L18 (-0.5, 6.6) -> (-0.5, 2.6)
  line L19 (-0.5, 6.6) -> (8.5, 2.6)
  point P0 (64, 2.6)
  point P1 (53, 5.9333)
  point P2 (1, 5.9333)
  dimension "d173" = 1.5
  dimension "d174" = 4
  dimension "d175" = 1.5
  dimension "d176" = 9
  dimension "d177" = 9
  constraints: 36 end point, 8 parallel, 4 horizontal, 4 perpendicular, 1 point on line
  measures "d173" distance of L2.end L3.end
  measures "d174" distance of L1.end L2.end
  measures "d175" distance of L7.end L8.end
  measures "d176" distance of L11.end L12.end
  measures "d177" distance of L17.end L16.end
extrude "Extrusion15" add sketch "Sketch17" against normal blind 10 contours L4 L19 L15 | L5 L10 L14
extrude "Extrusion16" add sketch "Sketch16" against normal blind 10 contours L18 L10 L0 | L14 L19 L9
sketch "Sketch18" plane through (10, -2.6, -21.9978) normal (0, 0, -1) x (-1, 0, 0)
  point P0 (10, 2.6)
sketch "Sketch19" plane through (10, -2.6, -21.9978) normal (0, 0, -1) x (-1, 0, 0)
  line L0 (-53, 2.6) -> (-53, 5.9333) projected
  line L1 (-53, 4.2667) -> (-45.6067, 4.2667)
  line L2 (-45.6067, 4.2667) -> (-1, 4.2667)
  line L3 (-1, 5.9333) -> (-1, 2.6) projected
  line L4 (-45.5, 2.6) -> (-53, 2.6) projected
  line L5 (-53, 4.2667) -> (-48, 4.2667)
  line L6 (-48, 4.2667) -> (-48, 2.6)
  line L7 (-48, 2.6) -> (-53, 2.6)
  line L8 (-53, 2.6) -> (-53, 4.2667)
  line L9 (-7.5, 2.6) -> (-4.5, 2.6) projected
  line L10 (-1, 4.2667) -> (-6, 4.2667)
  line L11 (-6, 4.2667) -> (-6, 2.6)
  line L12 (-6, 2.6) -> (-1, 2.6)
  line L13 (-1, 2.6) -> (-1, 4.2667)
  line L14 (-53, 4.2667) -> (-48, 2.6)
  line L15 (-1, 4.2667) -> (-6, 2.6)
  point P0 (10, 2.6)
  dimension "d182" = 5
  dimension "d183" = 5
  constraints: 24 end point, 4 parallel, 3 horizontal, 3 midpoint, 2 perpendicular, 1 point on line
  measures "d182" distance of L6.end L7.end
  measures "d183" distance of L12.end L11.end
extrude "Extrusion17" add sketch "Sketch19" along normal blind 45 contours L0 L14 L4 | L3 L12 L9 L15
fillet "Fillet1" radius 6.67 1 edges at (11, 3.3333, -16.9978)
fillet "Fillet2" radius 6.67 1 edges at (11, 3.3333, -69)
fillet "Fillet3" radius 6.67 1 edges at (63, 3.3333, -69)
fillet "Fillet4" radius 6.67 1 edges at (63, 3.3333, -16.9989)
fillet "Face Fillet19" radius 3 1 edges at (63, 1.6667, -42.9989)
fillet "Face Fillet20" radius 3 1 edges at (11, 1.6667, -42.9989)
fillet "Face Fillet21" radius 1.4 2 edges at (11.5663, 2.0748, -21.9978) (14.5257, 0.4914, -21.9978)
fillet "Face Fillet22" radius 1.4 2 edges at (11.5663, 2.0748, -64) (14.5257, 0.4914, -64)
fillet "Face Fillet23" radius 1.4 2 edges at (59.4743, 0.4914, -21.9978) (62.4337, 2.0748, -21.9978)
fillet "Face Fillet24" radius 1.4 2 edges at (62.4337, 2.0748, -64) (59.4743, 0.4914, -64)
fillet "Fillet5" radius 1.4 1 edges at (14.25, 0, -11.9978)
fillet "Fillet6" radius 1.4 2 edges at (59.25, 0, -11.9978) (63.5, 0, -12)
fillet "Fillet7" radius 1.4 1 edges at (59.75, 0, -74)
fillet "Fillet8" radius 1.4 1 edges at (14.25, 0, -74)
fillet "Fillet9" radius 1.4 2 edges at (64, 0.7, -74) (64, -1.3, -74)
fillet "Fillet10" radius 1.4 2 edges at (10, 0.7, -74) (10, -1.3, -74)
fillet "Fillet11" radius 1.4 1 edges at (10, -0.6, -11.9978)
fillet "Fillet12" radius 1.4 1 edges at (64, -0.6, -12)
body "Solid1"
